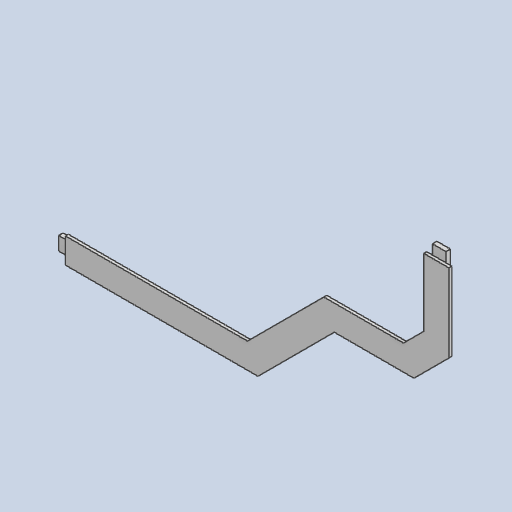
# Autodesk Inventor part: right_line
Saved by Autodesk Inventor 2022 (Build 260153000, 153)
## iProperties
Created: 2024-07-10
Part Number: right_line
Material: Типовые
Document SubType Name: Modeling
Designer: Капустяник Андрей
Density: 1 g/cm^3
Appearance: По умолчанию
Author: Капустяник Андрей
Autodesk Inventor part; units mm, degrees
ref_plane "YZ Plane" through (0, 0, 0) normal (1, 0, 0) x (0, 1, 0)
ref_plane "XZ Plane" through (0, 0, 0) normal (0, 1, 0) x (-1, 0, 0)
ref_plane "XY Plane" through (0, 0, 0) normal (0, 0, 1) x (1, 0, 0)
sketch "Эскиз1" plane through (0, 0, 0) normal (0, 0, 1) x (1, 0, 0)
  line L0 (-75.0711, -58) -> (-141.1512, -58) projected
  line L1 (-141.1512, -58) -> (-141.1512, -4.9289) projected
  line L2 (-141.1512, -4.9289) -> (-133.2223, 3) projected
  line L3 (-14, 3) -> (-133.2223, 3) projected
  line L4 (-14, 3) -> (-14, -24.0711) projected
  line L5 (-14, -24.0711) -> (-21.9289, -32) projected
  line L6 (-21.9289, -32) -> (-49.0711, -32) projected
  line L7 (-49.0711, -32) -> (-75.0711, -58) projected
  line L8 (-131.1512, -2) -> (-136.1512, -7) projected
  line L9 (-136.1512, -7) -> (-136.1512, -13.8712) projected
  line L10 (-136.1512, -13.8712) -> (-136.1512, -19.5281) projected
  line L11 (-136.1512, -19.5281) -> (-136.1512, -26.3992) projected
  line L12 (-136.1512, -26.3992) -> (-136.1512, -27) projected
  line L13 (-136.1512, -27) -> (-131.0951, -27) projected
  line L14 (-131.0951, -27) -> (-124.224, -27) projected
  line L15 (-124.224, -27) -> (-118.5671, -27) projected
  line L16 (-118.5671, -27) -> (-111.696, -27) projected
  line L17 (-111.696, -27) -> (-106.0391, -27) projected
  line L18 (-106.0391, -27) -> (-99.168, -27) projected
  line L19 (-99.168, -27) -> (-93.5111, -27) projected
  line L20 (-93.5111, -27) -> (-86.64, -27) projected
  line L21 (-86.64, -27) -> (-80.9831, -27) projected
  line L22 (-80.9831, -27) -> (-74.112, -27) projected
  line L23 (-74.112, -27) -> (-68.4551, -27) projected
  line L24 (-68.4551, -27) -> (-61.584, -27) projected
  line L25 (-61.584, -27) -> (-55.9271, -27) projected
  line L26 (-55.9271, -27) -> (-49.056, -27) projected
  line L27 (-49.056, -27) -> (-43.3991, -27) projected
  line L28 (-43.3991, -27) -> (-36.528, -27) projected
  line L29 (-36.528, -27) -> (-30.8711, -27) projected
  line L30 (-30.8711, -27) -> (-24, -27) projected
  line L31 (-24, -27) -> (-19, -22) projected
  line L32 (-19, -22) -> (-19, -15.1289) projected
  line L33 (-19, -15.1289) -> (-19, -9.472) projected
  line L34 (-19, -9.472) -> (-19, -2.6009) projected
  line L35 (-19, -2.6009) -> (-19, -2) projected
  line L36 (-19, -2) -> (-24.056, -2) projected
  line L37 (-24.056, -2) -> (-30.9271, -2) projected
  line L38 (-30.9271, -2) -> (-36.584, -2) projected
  line L39 (-36.584, -2) -> (-43.4551, -2) projected
  line L40 (-43.4551, -2) -> (-49.112, -2) projected
  line L41 (-49.112, -2) -> (-55.9831, -2) projected
  line L42 (-55.9831, -2) -> (-61.64, -2) projected
  line L43 (-61.64, -2) -> (-68.5111, -2) projected
  line L44 (-68.5111, -2) -> (-74.168, -2) projected
  line L45 (-74.168, -2) -> (-81.0391, -2) projected
  line L46 (-81.0391, -2) -> (-86.696, -2) projected
  line L47 (-86.696, -2) -> (-93.5671, -2) projected
  line L48 (-93.5671, -2) -> (-99.224, -2) projected
  line L49 (-99.224, -2) -> (-106.0951, -2) projected
  line L50 (-106.0951, -2) -> (-111.752, -2) projected
  line L51 (-111.752, -2) -> (-118.6231, -2) projected
  line L52 (-118.6231, -2) -> (-124.28, -2) projected
  line L53 (-124.28, -2) -> (-131.1512, -2) projected
  line L54 (-141.1512, -69.9) -> (-42.8584, -69.9) projected
  line L55 (-141.1512, -63) -> (-141.1512, -69.9) projected
  line L56 (-141.1512, -63) -> (-73, -63) projected
  line L57 (-73, -63) -> (-47, -37) projected
  line L58 (-47, -37) -> (-19.8579, -37) projected
  line L59 (-19.8579, -37) -> (-9, -26.1421) projected
  line L60 (-9, -26.1421) -> (-9, 3) projected
  line L61 (-9, 3) -> (-2, 3) projected
  line L62 (-2, -29.0416) -> (-2, 3) projected
  line L63 (-42.8584, -69.9) -> (-2, -29.0416) projected
  line L64 (-73.0828, -62.8) -> (-141.3512, -62.8)
  line L65 (-141.3512, -62.8) -> (-141.3512, -70.1)
  line L66 (-141.3512, -70.1) -> (-42.7755, -70.1)
  line L67 (-42.7755, -70.1) -> (-1.8, -29.1245)
  line L68 (-1.8, -29.1245) -> (-1.8, 3.2)
  line L69 (-1.8, 3.2) -> (-9.2, 3.2)
  line L70 (-9.2, 3.2) -> (-9.2, -26.0593)
  line L71 (-9.2, -26.0593) -> (-19.9407, -36.8)
  line L72 (-19.9407, -36.8) -> (-47.0828, -36.8)
  line L73 (-47.0828, -36.8) -> (-73.0828, -62.8)
  line L74 (-141.3512, -58.2) -> (-74.9882, -58.2)
  line L75 (-74.9882, -58.2) -> (-48.9882, -32.2)
  line L76 (-48.9882, -32.2) -> (-21.8461, -32.2)
  line L77 (-21.8461, -32.2) -> (-13.8, -24.1539)
  line L78 (-13.8, -24.1539) -> (-13.8, 3.2)
  line L79 (-13.8, 3.2) -> (-133.3051, 3.2)
  line L80 (-133.3051, 3.2) -> (-141.3512, -4.8461)
  line L81 (-141.3512, -4.8461) -> (-141.3512, -58.2)
  line L82 (-141.1512, -58) -> (-141.1512, -66.7) projected
  line L83 (-5.3, 3) -> (-14, 3) projected
  line L84 (-44.9289, -42) -> (-65.9289, -63) projected
  line L85 (-65.9289, -63) -> (-45.8579, -63) projected
  line L86 (-45.8579, -63) -> (-24.8579, -42) projected
  line L87 (-24.8579, -42) -> (-44.9289, -42) projected
  point P0 (-9.2, 3)
  point P1 (-13.8, 3)
  point P2 (-141.1512, -58.2)
  point P3 (-141.1512, -62.8)
  dimension "d10" = 0.2
  dimension "d11" = 0.2
  constraints: 36 end point, 16 other
  measures "d10" distance between parallel lines of L56 L64
  measures "d11" distance between parallel lines of L0 L74
extrude "Выдавливание1" add sketch "Эскиз1" against normal blind 1.5 contours L74 L75 L76 L77 L78 L83 L70 L71 L72 L73 L64 L82
sketch "Эскиз2" plane through (0, 0, 0) normal (0, 0, 1) x (1, 0, 0)
  line L0 (-19.9407, -36.8) -> (-47.0828, -36.8) projected
  line L1 (-47.0828, -36.8) -> (-73.0828, -62.8) projected
  line L2 (-73.0828, -62.8) -> (-141.1512, -62.8) projected
  line L3 (-141.1512, -62.8) -> (-141.1512, -58.2) projected
  line L4 (-141.1512, -58.2) -> (-74.9882, -58.2) projected
  line L5 (-74.9882, -58.2) -> (-48.9882, -32.2) projected
  line L6 (-48.9882, -32.2) -> (-21.8461, -32.2) projected
  line L7 (-21.8461, -32.2) -> (-13.8, -24.1539) projected
  line L8 (-13.8, -24.1539) -> (-13.8, 3) projected
  line L9 (-13.8, 3) -> (-9.2, 3) projected
  line L10 (-9.2, 3) -> (-9.2, -26.0593) projected
  line L11 (-9.2, -26.0593) -> (-19.9407, -36.8) projected
  line L12 (-75.8167, -56.2) -> (-143.1512, -56.2)
  line L13 (-143.1512, -56.2) -> (-143.1512, -64.8)
  line L14 (-143.1512, -64.8) -> (-72.2544, -64.8)
  line L15 (-72.2544, -64.8) -> (-46.2544, -38.8)
  line L16 (-46.2544, -38.8) -> (-19.1123, -38.8)
  line L17 (-19.1123, -38.8) -> (-7.2, -26.8877)
  line L18 (-7.2, -26.8877) -> (-7.2, 5)
  line L19 (-7.2, 5) -> (-15.8, 5)
  line L20 (-15.8, 5) -> (-15.8, -23.3255)
  line L21 (-15.8, -23.3255) -> (-22.6745, -30.2)
  line L22 (-22.6745, -30.2) -> (-49.8167, -30.2)
  line L23 (-49.8167, -30.2) -> (-75.8167, -56.2)
  line L24 (-138.1512, -66.9) -> (-138.1512, -63) projected
  line L25 (-14, 0) -> (-5.3, 0) projected
  line L26 (-7.2, 0) -> (-7.2, -0.3)
  line L27 (-7.2, -0.3) -> (-15.8, -0.3)
  line L28 (-138.1512, -64.8) -> (-137.8512, -64.8)
  line L29 (-137.8512, -64.8) -> (-137.8512, -56.2)
  dimension "d12" = 2
  dimension "d13" = 0.3
  dimension "d14" = 0.3
  constraints: 32 end point, 8 point on line, 2 perpendicular, 11 other
  measures "d12" distance between parallel lines of L4 L12
  measures "d13" distance of L26.start L26.end
  measures "d14" distance of L28.start L28.end
extrude "Выдавливание2" add sketch "Эскиз2" along normal blind 1 contours L11 L10 L27 L18 L17 L16 L15 L14 L29 L2 L1 L0 | L0 L1 L2 L29 L4 L5 L6 L7 L8 L27 L10 L11 | L8 L7 L6 L5 L4 L29 L12 L23 L22 L21 L20 L27
